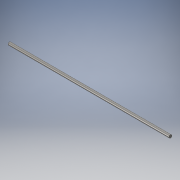
# Autodesk Inventor part: X-axis axle
Saved by Autodesk Inventor 2018 (Build 220112000, 112)
## iProperties
Created: 2013-10-26
Part Number: X-axis axle
Material: Steel, Carbon
Document SubType Name: Modeling
Designer: Gabriel Smolnycki
Mass: 40.8456 g
Surface Area: 42.0188 cm^2
Volume: 5.20326 cm^3
Density: 7.85 g/cm^3
Appearance: Semi-Polished
Sending System: SolidWorks 2017
Last Author: Gabriel Smolnycki
Last Saved: 2017-09-14
Author: Gabriel Smolnycki
Autodesk Inventor part; units mm, degrees
ref_plane "XZ Plane" through (0, 0, 0) normal (0, 1, 0) x (-1, 0, 0)
ref_plane "XY Plane" through (0, 0, 0) normal (0, 0, 1) x (1, 0, 0)
ref_plane "Work Plane1" through (265, 0, 0) normal (1, 0, 0) x (0, 1, 0)
sketch "Sketch1" plane through (265, 0, 0) normal (1, 0, 0) x (0, 1, 0)
  circle A0 centre (0, 0) radius 2.5
  constraints: 1 centre point
extrude "Extrusion1" add sketch "Sketch1" against normal blind 265
body "Solid3"
